Autodesk Fusion 360 part; units mm, degrees
note: some values were not read from the file. Set by a fixed rule: which face or edge a step refers to.
(part 2 of 2)
fillet "Fillet1''" radius 1 16 edges at (63, 40.5, 78) (-63, 40.5, 78) (0, -2, 78) (63, -2, -10) (63, 40.5, -98) (-63, 40.5, -98) (0, -2, -98) (-63, -2, -10) (-63, 83, -10) (0, 83, 78) (63, 83, -10) (52.5, 83, -98) (29.75, 83, -98) (0, 83, -98) (-29.75, 83, -98) (-52.5, 83, -98) on bodies 1 in component "Box"
fillet "Fillet2'" radius 0.5 16 edges at (42, 76.9087, -101.118) (42, 86.3035, -102.6562) (34, 86.3035, -102.6562) (34, 76.9087, -101.118) (17.5, 86.3035, -102.6562) (17.5, 76.9087, -101.118) (25.5, 76.9087, -101.118) (25.5, 86.3035, -102.6562) (-17.5, 76.9087, -101.118) (-17.5, 86.3035, -102.6562) (-25.5, 86.3035, -102.6562) (-25.5, 76.9087, -101.118) (-34, 76.9087, -101.118) (-34, 86.3035, -102.6562) (-42, 86.3035, -102.6562) (-42, 76.9087, -101.118) on bodies 1 in component "Box"
fillet "Fillet1'''" radius 1 12 edges at (0, 86, -10) (-63, 84.5, -10) (-63, 86, 34) (-63, 83, 34) (0, 83, -10) (63, 86, 34) (63, 84.5, -10) (63, 83, 34) (63, 84.5, 78) (0, 83, 78) (0, 86, 78) (-63, 84.5, 78) on bodies 6 in component "Lid"
fillet "Fillet2''" radius 0.5 4 edges at (61.297, 86, 74.5848) (61.297, 86, 1.0848) (-55.703, 86, 1.0848) (-55.703, 86, 74.5848) on bodies 6 in component "Lid"
fillet "Fillet3" radius 1 10 edges at (63, 86, -54.5) (63, 84.5, -11) (0, 83, -11) (63, 83, -54.5) (0, 86, -11) (63, 84.5, -98) (-63, 84.5, -98) (-63, 83, -54.5) (-63, 86, -54.5) (-63, 84.5, -11) on bodies 7 in component "Lid"
sketch "Sketch10 (2)" plane through (0, 0, -98) normal (0, 0, -1) x (-1, 0, 0) in component "Box"
  line L0 (34, 82) -> (25.5, 82)
  line L1 (25.5, 82) -> (25.5, 73.8018)
  ellipse E0 centre (25, 73.8018) end of major axis (25, 73) minor radius 0.5 (25, 73) -> (25.5, 73.8018) ccw
  line L2 (25, 73) -> (18, 73)
  ellipse E1 centre (18, 73.8018) end of major axis (18, 73) minor radius 0.5 (17.5, 73.8018) -> (18, 73) ccw
  line L3 (17.5, 73.8018) -> (17.5, 82)
  line L4 (17.5, 82) -> (-17.5, 82)
  line L5 (-17.5, 82) -> (-17.5, 73.8018)
  ellipse E2 centre (-18, 73.8018) end of major axis (-18, 73) minor radius 0.5 (-18, 73) -> (-17.5, 73.8018) ccw
  line L6 (-18, 73) -> (-25, 73)
  ellipse E3 centre (-25, 73.8018) end of major axis (-25, 73) minor radius 0.5 (-25.5, 73.8018) -> (-25, 73) ccw
  line L7 (-25.5, 73.8018) -> (-25.5, 82)
  line L8 (-25.5, 82) -> (-34, 82)
  line L9 (-34, 82) -> (-34, 73.8018)
  ellipse E4 centre (-34.5, 73.8018) end of major axis (-34.5, 73) minor radius 0.5 (-34.5, 73) -> (-34, 73.8018) ccw
  line L10 (-34.5, 73) -> (-41.5, 73)
  ellipse E5 centre (-41.5, 73.8018) end of major axis (-41.5, 73) minor radius 0.5 (-42, 73.8018) -> (-41.5, 73) ccw
  line L11 (-42, 73.8018) -> (-42, 82)
  line L12 (-42, 82) -> (-62, 82)
  line L13 (-62, 82) -> (-62, -1)
  line L14 (-62, -1) -> (62, -1)
  line L15 (62, -1) -> (62, 82)
  line L16 (62, 82) -> (42, 82)
  line L17 (42, 82) -> (42, 73.8018)
  ellipse E6 centre (41.5, 73.8018) end of major axis (41.5, 73) minor radius 0.5 (41.5, 73) -> (42, 73.8018) ccw
  line L18 (41.5, 73) -> (34.5, 73)
  ellipse E7 centre (34.5, 73.8018) end of major axis (34.5, 73) minor radius 0.5 (34, 73.8018) -> (34.5, 73) ccw
  line L19 (34, 73.8018) -> (34, 82)
  line L20 (0, 0) -> (0, 14)
  line L21 (-11.5372, 14) -> (-11.5372, 29)
  line L22 (-11.5372, 29) -> (-46.5372, 29)
  line L23 (-46.5372, 29) -> (-46.5372, 14)
  line L24 (-46.5372, 14) -> (-11.5372, 14)
  line L25 (-46.5372, 14) -> (-11.5372, 14)
  line L26 (-11.5372, 29) -> (-11.5372, 14) construction
  line L27 (-46.5372, 29) -> (-46.5372, 14)
  line L28 (-46.5372, 14) -> (-11.5372, 14)
  line L29 (-11.5372, 29) -> (-46.5372, 29)
  line L30 (-11.5372, 14) -> (-11.5372, 29)
  line L31 (-46.5372, 29) -> (-46.5372, 14)
  line L32 (-11.5372, 14) -> (-46.5372, 14)
  dimension "d395" = 14
  dimension "d396" = 15
  dimension "d397" = 35
  constraint coincident L20.start origin
  constraint perpendicular L14 L20
  constraint perpendicular L21 L22
  measures "d395" distance of L20.start L20.end
  measures "d396" distance of L21.start L21.end
  measures "d397" distance of L21.end L22.end
extrude "Extrude14" cut sketch "Sketch10 (2)" against normal up to surface (3 mm away) contours L21 L22 L23 L24 L25 L27 L28 L29 L30 L31 L32 bodies 1 in component "Box"
fillet "Fillet3'" radius 0.5 4 edges at (46.5372, 21.5, -98) (29.0372, 29, -98) (29.0372, 14, -98) (11.5372, 21.5, -98) on bodies 1 in component "Box"
fillet "Fillet1''''" radius 0.5 1 edges at (44, 82.096, -99.1692) on bodies 8 in component "Hinge_pipe"
fillet "Fillet1'''''" radius 0.5 1 edges at (-49, 82.096, -103.8308) on bodies 9 in component "Pipe_end"
fillet "Fillet1''''''" radius 0.5 23 edges at (22, 41, -12) (27, 41, -12) (22, 30, 9.5) (27, 30, 9.5) (24.5, 30, -12) (24.5, 52, -12) (24.5, 52, -18) (27, 29, -18) (22, 29, -18) (19.3308, 8, -15.904) (34.3308, 8, -15.904) (24.5, 30, 31) (27, 41, 31) (22, 41, 31) (24.5, 52, 31) (22, 52, 34) (27, 52, 34) (27, 52, -15) (22, 52, -15) (22, 29, 37) (27, 29, 37) (19.3308, 8, 33.096) (34.3308, 8, 33.096) on bodies 3 in component "Switch_servo_mount"
fillet "Fillet1'''''''" radius 0.5 24 edges at (-36.5, 78, -40.5) (-39, 78, -43.25) (-34, 78, -43.25) (-36.5, 78, -46) (-36.5, 78, -75.5) (-34, 70.25, -46) (-39, 70.25, -46) (-36.5, 62.5, -46) (-34, 62.5, -60.75) (-39, 62.5, -60.75) (-36.5, 78, -81) (-34, 78, -78.25) (-39, 78, -78.25) (-36.5, 62.5, -75.5) (-34, 70.25, -75.5) (-39, 70.25, -75.5) (-39, 42, -40.5) (-34, 42, -40.5) (-34, 42, -81) (-39, 42, -81) (-41.6692, 8, -78.904) (-41.6692, 8, -44.404) (-26.6692, 8, -44.404) (-26.6692, 8, -78.904) on bodies 2 in component "Lid_servo_mount"
extrude "Extrude6'" [suppressed] in component "Box"
extrude "Extrude4'''''" [suppressed] in component "Box"
extrude "Extrude3'''''" [suppressed] in component "Box"
sketch "Sketch4 (3)" plane through (22, 0, 0) normal (-1, 0, 0) x (0, 0, 1) in component "Box"
  line L0 (-18, 3) -> (37, 3)
  line L1 (37, 3) -> (37, 78)
  line L2 (37, 78) -> (-18, 78)
  line L3 (-18, 78) -> (-18, 3)
  line L4 (34, 78) -> (34, 57) construction
  line L5 (-15, 78) -> (-15, 57) construction
  line L6 (-15, 57) -> (34, 57) construction
  line L7 (-15, 67.5) -> (34, 67.5)
  circle A0 centre (-15, 72.5) radius 0.85
  circle A1 centre (-15, 62.5) radius 0.85
  circle A2 centre (34, 62.5) radius 0.85
  circle A3 centre (34, 72.5) radius 0.85
  line L8 (-12, 78) -> (-12, 57)
  line L9 (31, 78) -> (31, 57)
  circle A4 centre (0, 67.5) radius 2.5
  dimension "d58" = 3
  dimension "d59" = 21
  dimension "d60" = 3
  dimension "d61" = 1.7
  dimension "d62" = 1.7
  dimension "d63" = 1.7
  dimension "d64" = 1.7
  dimension "d71" = 3
  dimension "d72" = 3
  dimension "d110" = 5
  dimension "d111" = 15
  dimension "d112" = 10.5
  constraint coincident L2 L4.start
  constraint perpendicular L2 L4
  constraint coincident L2 L5.start
  constraint perpendicular L2 L5
  constraint midpoint L5 L7.start
  constraint midpoint L4 L7.end
  constraint perpendicular L4 L7
  constraint coincident L5 A0.centre
  constraint coincident L5 A1.centre
  constraint coincident L4 A2.centre
  constraint coincident L4 A3.centre
  constraint coincident L2 L8.start
  constraint coincident L6 L8.end
  constraint perpendicular L6 L8
  constraint coincident L2 L9.start
  constraint coincident L6 L9.end
  constraint perpendicular L6 L9
  constraint coincident L7 A4.centre
  measures "d58" distance of L1 L4
  measures "d59" distance of L5.start L5.end
  measures "d60" distance of L3 L5
  measures "d61" diameter of A0
  measures "d62" diameter of A1
  measures "d63" diameter of A2
  measures "d64" diameter of A3
  measures "d71" distance of L5 L8
  measures "d72" distance of L4 L9
  measures "d110" diameter of A4
  measures "d111" distance of L5 A4.centre
  measures "d112" distance of L6 A4.centre
move_face "OffsetFaces1''" [suppressed] in component "Box"
extrude "Extrude5'''" [suppressed] in component "Box"
sketch "Sketch5 (3)" plane through (-39, 0, 0) normal (-1, 0, 0) x (0, 0, 1) in component "Box"
  line L0 (-81, 3) -> (-40.5, 3)
  line L1 (-40.5, 3) -> (-40.5, 78)
  line L2 (-40.5, 78) -> (-81, 78)
  line L3 (-81, 78) -> (-81, 3)
  line L4 (-78, 78) -> (-78, 63) construction
  line L5 (-43.5, 78) -> (-43.5, 63) construction
  line L6 (-75, 78) -> (-75, 63)
  line L7 (-46.5, 78) -> (-46.5, 63)
  circle A0 centre (-43.5, 70) radius 1
  circle A1 centre (-78, 70) radius 1
  dimension "d86" = 15
  dimension "d87" = 3
  dimension "d88" = 15
  dimension "d89" = 3
  dimension "d90" = 15
  dimension "d91" = 15
  dimension "d92" = 3
  dimension "d93" = 3
  dimension "d94" = 2
  dimension "d95" = 2
  dimension "d96" = 7
  dimension "d97" = 7
  constraint coincident L2 L4.start
  constraint perpendicular L2 L4
  constraint coincident L2 L5.start
  constraint perpendicular L2 L5
  constraint coincident L2 L6.start
  constraint perpendicular L2 L6
  constraint coincident L2 L7.start
  constraint perpendicular L2 L7
  constraint coincident L5 A0.centre
  constraint coincident L4 A1.centre
  measures "d86" distance of L4.start L4.end
  measures "d87" distance of L3 L4
  measures "d88" distance of L5.start L5.end
  measures "d89" distance of L1 L5
  measures "d90" distance of L6.start L6.end
  measures "d91" distance of L7.start L7.end
  measures "d92" distance of L4 L6
  measures "d93" distance of L5 L7
  measures "d94" diameter of A0
  measures "d95" diameter of A1
  measures "d96" distance of L4.end A1.centre
  measures "d97" distance of L5.end A0.centre
extrude "Extrude7'" [suppressed] in component "Box"
extrude "Extrude8'" [suppressed] in component "Box"
sketch "Sketch1 (7)" plane through (0, 83, 0) normal (0, 1, 0) x (-1, 0, 0) in component "Lid"
  line L0 (-60, -95) -> (-60, 75)
  line L1 (-60, 75) -> (60, 75)
  line L2 (60, 75) -> (60, -95)
  line L3 (60, -95) -> (-60, -95)
  line L4 (-63, 78) -> (-63, -98)
  line L5 (-63, -98) -> (63, -98)
  line L6 (63, -98) -> (63, 78)
  line L7 (63, 78) -> (-63, 78)
  line L8 (63, 78) -> (-63, 78)
  line L9 (-63, 78) -> (-63, -10)
  line L10 (-63, -10) -> (63, -10)
  line L11 (63, -10) -> (63, 78)
  dimension "d102" = 126
  dimension "d103" = 88
  constraint horizontal L8
  constraint vertical L9
  constraint horizontal L10
  constraint vertical L11
  constraint coincident L6.end L7.start
  measures "d102" distance of L6.end L4.start
  measures "d103" distance of L6.end L10.end
extrude "Extrude1''''''" [suppressed] in component "Lid"
sketch "Sketch2 (8)" plane through (0, 86, 0) normal (0, 1, 0) x (-1, 0, 0) in component "Lid"
  line L0 (63, -10) -> (63, 78)
  line L1 (63, 78) -> (-63, 78)
  line L2 (-63, 78) -> (-63, -10)
  line L3 (-63, -10) -> (63, -10)
  circle A0 centre (0, 0) radius 3.1
  dimension "d106" = 6.2
  constraint coincident A0.centre origin
  measures "d106" diameter of A0
extrude "Extrude2''''''" [suppressed] in component "Lid"
sketch "Sketch1 (8)" plane through (0, 0, 0) normal (1, 0, 0) x (0, 0, -1) in component "Switch_finger"
sketch "Sketch6 (2)" plane through (22, 0, 0) normal (-1, 0, 0) x (0, 0, 1) in component "Box"
  line L0 (-18, 3) -> (37, 3)
  line L1 (37, 3) -> (37, 58)
  line L2 (37, 58) -> (-18, 58)
  line L3 (-18, 58) -> (-18, 3)
move_face "OffsetFaces3" [suppressed] in component "Box"
move_face "OffsetFaces2" [suppressed] in component "Box"
component "Box" placed x (1, 0, 0) y (0, 1, 0) z (0, 0, 1) at (0, 0, 0)
component "Lid" placed x (1, 0, 0) y (0, 1, 0) z (0, 0, 1) at (0, 0, 0)
component "Hinge_pipe" placed x (1, 0, 0) y (0, 1, 0) z (0, 0, 1) at (0, 0, 0)
component "Pipe_end" placed x (1, 0, 0) y (0, 1, 0) z (0, 0, 1) at (0, 0, 0)
component "Switch_servo_mount" placed x (1, 0, 0) y (0, 1, 0) z (0, 0, 1) at (0, 0, 0)
component "Lid_servo_mount" placed x (1, 0, 0) y (0, 1, 0) z (0, 0, 1) at (0, 0, 0)
component "Finger_switch" placed x (1, 0, 0) y (0, 1, 0) z (0, 0, 1) at (0, 0, 0)
component "Finger_lid" placed x (1, 0, 0) y (0, 1, 0) z (0, 0, 1) at (0, 0, 0)
hidden bodies 6 7
equation "Box_width = 120 mm"
equation "box_height = 80 mm"
equation "box_thickness = 3 mm"
equation "screw_hole_25 = 2.1 mm"
equation "screw_hole_lid_servo = 2 mm"
equation "screw_hole_switch_servo = 1.7 mm"
equation "cb_length = 56 mm"
equation "cb_width = 36 mm"
equation "x_servo_to_switch = 19.5 mm + 2.5 mm"
equation "switch_servo_hole_z = 49 mm"
equation "switch_servo_hole_y = 10 mm"
equation "switch_hole = 6.2 mm"
equation "hinge_hole_d = 3 mm"
equation "lid_servo_hole_z = 34.5 mm"
equation "cb_mount_height = 12 mm"
equation "lid_servo_mount_distance_from_wall = 21 mm"
equation "servo_mount_thickness = 5 mm"
equation "cb_mount_outer_d = 5 mm"
equation "box_length = 170 mm"
equation "d20 = Box_width"
equation "d21 = box_length"
equation "d22 = box_thickness"
equation "switch_servo_axis = 15 mm"
equation "lid_servo_axis = 11 mm"
equation "d26 = box_thickness"
equation "d27 = box_thickness"
equation "d28 = box_length + 2 * box_thickness"
equation "d29 = Box_width + 2 * box_thickness"
equation "d30 = box_length + 2 * box_thickness"
equation "d31 = Box_width + 2 * box_thickness"
equation "d34 = Box_width"
equation "d35 = box_length"
equation "d36 = cb_width"
equation "d37 = cb_length"
equation "d44 = screw_hole_25"
equation "d45 = screw_hole_25"
equation "d46 = screw_hole_25"
equation "d47 = screw_hole_25"
equation "d50 = x_servo_to_switch"
equation "d51 = switch_servo_axis + 3 mm"
equation "d52 = servo_mount_thickness"
equation "d53 = switch_servo_hole_z + 6 mm"
equation "d54 = servo_mount_thickness"
equation "d55 = box_height - 5 mm"
equation "d61 = screw_hole_switch_servo"
equation "d62 = screw_hole_switch_servo"
equation "d63 = screw_hole_switch_servo"
equation "d64 = screw_hole_switch_servo"
equation "lid_servo_mount_z_distance_from_wall = 17 mm"
equation "d76 = servo_mount_thickness"
equation "d77 = lid_servo_mount_z_distance_from_wall"
equation "d78 = lid_servo_hole_z"
equation "d79 = lid_servo_mount_distance_from_wall"
equation "d84 = box_height - 5 mm"
equation "d94 = screw_hole_lid_servo"
equation "d95 = screw_hole_lid_servo"
equation "d100 = box_height"
equation "d102 = ( Box_width + 2 * box_thickness )"
equation "d103 = ( box_length + 2 * box_thickness ) / 2"
equation "d104 = box_thickness"
equation "d106 = switch_hole"
equation "d114 = -box_height"
equation "d131 = screw_hole_25"
equation "d132 = screw_hole_25"
equation "d133 = screw_hole_25"
equation "d134 = screw_hole_25"
equation "d135 = box_height - 1 mm - 30 mm"
equation "d150 = screw_hole_switch_servo"
equation "d151 = screw_hole_switch_servo"
equation "d152 = screw_hole_switch_servo"
equation "d153 = screw_hole_switch_servo"
equation "d161 = switch_servo_axis"
equation "d164 = box_height + box_thickness + 14 mm"
equation "d165 = box_height + box_thickness"
equation "d166 = ( box_length + 2 * box_thickness ) / 2"
equation "d167 = box_height + box_thickness"
equation "d182 = screw_hole_25"
equation "d184 = screw_hole_25"
equation "d214 = screw_hole_25"
equation "d215 = screw_hole_25"
equation "d216 = screw_hole_25"
equation "d217 = screw_hole_25"
equation "d220 = box_height - 5 mm"
equation "d232 = screw_hole_lid_servo"
equation "d233 = screw_hole_lid_servo"
equation "d239 = screw_hole_25"
equation "d240 = screw_hole_25"
equation "d241 = screw_hole_25"
equation "d242 = screw_hole_25"
equation "d243 = screw_hole_25"
equation "d244 = screw_hole_25"
equation "d245 = screw_hole_25"
equation "d246 = screw_hole_25"
equation "d251 = box_height"
equation "d261 = screw_hole_25"
equation "d263 = screw_hole_25"
equation "d268 = box_height"
equation "d270 = Box_width + 2 * box_thickness"
equation "d271 = ( box_length + 2 * box_thickness ) / 2"
equation "d272 = box_thickness"
equation "d274 = switch_hole"
equation "d281 = screw_hole_25"
equation "d282 = screw_hole_25"
equation "d283 = screw_hole_25"
equation "d284 = screw_hole_25"
equation "d300 = 3 mm + 1.5 mm"
equation "d301 = 3 mm + 1.5 mm"
equation "d308 = screw_hole_25"
equation "d309 = screw_hole_25"
equation "d310 = screw_hole_25"
equation "d311 = screw_hole_25"
equation "d320 = Box_width + 2 * box_thickness"
equation "d321 = box_length / 2 + 3 mm - 1 mm"
equation "d322 = box_thickness"
equation "d341 = ( ( -126 / 2 ) * 1 mm ) + 3.5 mm"
